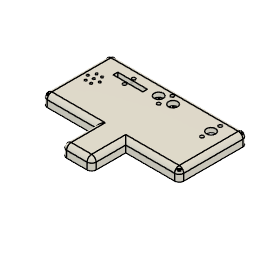
ControllerTopHalf (Autodesk Fusion 360 design; units mm, degrees)
part number: 2026-04-19-10-42-28-781
Autodesk Fusion 360 part; units mm, degrees
sketch "Sketch1" plane through (0, 0, 0) normal (0, 1, 0) x (1, 0, 0)
  line L0 (0, 0) -> (300, 0)
  line L1 (300, 0) -> (300, -150)
  line L2 (300, -150) -> (0, -150)
  line L3 (0, -150) -> (0, 0)
  line L4 (150, -150) -> (117.5, -150)
  line L5 (150, -150) -> (182.5, -150)
  line L6 (117.5, -150) -> (117.5, -225)
  line L7 (182.5, -150) -> (182.5, -225)
  line L8 (117.5, -225) -> (182.5, -225)
  dimension "d1" = 300
  dimension "d2" = 150
  dimension "d3" = 32.5
  dimension "d4" = 32.5
  dimension "d5" = 75
  dimension "d6" = 75
  constraint horizontal L0
  constraint vertical L1
  constraint horizontal L2
  constraint vertical L3
  constraint coincident L0.start L3.end
  constraint midpoint L2 L4.start
  constraint parallel L2 L4
  constraint parallel L2 L5
  constraint perpendicular L2 L6
  constraint perpendicular L2 L7
  measures "d1" distance of L0.start L0.end
  measures "d2" distance of L0.start L2.end
  measures "d3" distance of L4.start L4.end
  measures "d4" distance of L4.start L5.end
  measures "d5" distance of L4.end L6.end
  measures "d6" distance of L5.end L7.end
extrude "Extrude1" add sketch "Sketch1" along normal blind 25
fillet "Fillet1" radius 10 6 edges at (0, 12.5, 0) (0, 12.5, 150) (117.5, 12.5, 225) (182.5, 12.5, 225) (300, 12.5, 150) (300, 12.5, 0) 1 faces at (139.1667, 25, 50)
shell "Shell1" thickness 10 removed faces 1 at (139.1667, 0, 50)
sketch "Sketch2" plane through (0, 25, 0) normal (0, 1, 0) x (-1, 0, 0)
  line L0 (-127.5, 215) -> (-172.5, 215)
  line L1 (-172.5, 215) -> (-172.5, 140)
  line L2 (-172.5, 140) -> (-290, 140)
  line L3 (-290, 140) -> (-290, 10)
  line L4 (-290, 10) -> (-10, 10)
  line L5 (-10, 10) -> (-10, 140)
  line L6 (-10, 140) -> (-127.5, 140)
  line L7 (-127.5, 140) -> (-127.5, 215)
  circle A0 centre (-24.9278, 56.5112) radius 5
  circle A1 centre (-36.9278, 56.5112) radius 5
  circle A2 centre (-17.9278, 68.5112) radius 5
  circle A3 centre (-30.9278, 68.5112) radius 5
  circle A4 centre (-43.9278, 68.5112) radius 5
  circle A5 centre (-24.9278, 80.5112) radius 5
  circle A6 centre (-36.9278, 80.5112) radius 5
  dimension "d12" = 10
  dimension "d13" = 12
  dimension "d14" = 10
  dimension "d17" = 10
  dimension "d19" = 10
  dimension "d22" = 10
  dimension "d25" = 10
  dimension "d26" = 10
  measures "d12" diameter of A0
  measures "d13" distance of A0.centre A1.centre
  measures "d14" diameter of A1
  measures "d17" diameter of A2
  measures "d19" diameter of A3
  measures "d22" diameter of A4
  measures "d25" diameter of A5
  measures "d26" diameter of A6
hole "Hole1" at (17.9278, 25, 68.5112) at (24.9278, 25, 56.5112) at (30.9278, 25, 68.5112) at (36.9278, 25, 56.5112) at (43.9278, 25, 68.5112) at (36.9278, 25, 80.5112) at (24.9278, 25, 80.5112) direction (0, -1, 0) diameter 5 depth 16 tip angle 180
sketch "Sketch3" plane through (0, 25, 0) normal (0, 1, 0) x (-1, 0, 0)
  circle A0 centre (-36.9278, 80.5112) radius 2.5
  circle A1 centre (-36.9278, 56.5112) radius 2.5
  circle A2 centre (-24.9278, 56.5112) radius 2.5
  circle A3 centre (-17.9278, 68.5112) radius 2.5
  circle A4 centre (-30.9278, 68.5112) radius 2.5
  circle A5 centre (-43.9278, 68.5112) radius 2.5
  circle A6 centre (-24.9278, 80.5112) radius 2.5
  line L0 (-127.5, 215) -> (-172.5, 215)
  line L1 (-172.5, 215) -> (-172.5, 140)
  line L2 (-172.5, 140) -> (-290, 140)
  line L3 (-290, 140) -> (-290, 10)
  line L4 (-290, 10) -> (-10, 10)
  line L5 (-10, 10) -> (-10, 140)
  line L6 (-10, 140) -> (-127.5, 140)
  line L7 (-127.5, 140) -> (-127.5, 215)
  circle A7 centre (-260, 40) radius 10
  line L8 (-45, 30) -> (-110, 30)
  line L9 (-110, 30) -> (-110, 40)
  line L10 (-110, 40) -> (-45, 40)
  line L11 (-45, 40) -> (-45, 30)
  dimension "d30" = 20
  constraint horizontal L8
  constraint vertical L9
  constraint horizontal L10
  constraint vertical L11
  measures "d30" diameter of A7
extrude "Extrude2" cut sketch "Sketch3" against normal blind 50 contours A7 | L8 L9 L10 L11
sketch "Sketch4" plane through (0, 25, 0) normal (0, 1, 0) x (-1, 0, 0)
  line L0 (-110, 30) -> (-110, 40)
  line L1 (-110, 40) -> (-45, 40)
  line L2 (-45, 40) -> (-45, 30)
  line L3 (-45, 30) -> (-110, 30)
  circle A0 centre (-260, 40) radius 10
  circle A1 centre (-36.9278, 80.5112) radius 2.5
  circle A2 centre (-36.9278, 56.5112) radius 2.5
  circle A3 centre (-24.9278, 56.5112) radius 2.5
  circle A4 centre (-17.9278, 68.5112) radius 2.5
  circle A5 centre (-30.9278, 68.5112) radius 2.5
  circle A6 centre (-43.9278, 68.5112) radius 2.5
  circle A7 centre (-24.9278, 80.5112) radius 2.5
  line L4 (-127.5, 215) -> (-172.5, 215)
  line L5 (-172.5, 215) -> (-172.5, 140)
  line L6 (-172.5, 140) -> (-290, 140)
  line L7 (-290, 140) -> (-290, 10)
  line L8 (-290, 10) -> (-10, 10)
  line L9 (-10, 10) -> (-10, 140)
  line L10 (-10, 140) -> (-127.5, 140)
  line L11 (-127.5, 140) -> (-127.5, 215)
  circle A8 centre (-135, 30) radius 10
  line L12 (-172.5, 140) -> (-62.5, 140) construction
  circle A9 centre (-166.743, 30.1508) radius 10
  dimension "d33" = 20
  dimension "d36" = 20
  constraint horizontal L12
  constraint coincident L5.end L6.start
  measures "d33" diameter of A8
  measures "d36" diameter of A9
extrude "Extrude3" cut sketch "Sketch4" against normal blind 65 contours A8 | A9
sketch "Sketch5" plane through (0, 25, 0) normal (0, 1, 0) x (-1, 0, 0)
  circle A0 centre (-135, 30) radius 10
  circle A1 centre (-166.743, 30.1508) radius 10
  line L0 (-110, 30) -> (-110, 40)
  line L1 (-110, 40) -> (-45, 40)
  line L2 (-45, 40) -> (-45, 30)
  line L3 (-45, 30) -> (-110, 30)
  circle A2 centre (-260, 40) radius 10
  circle A3 centre (-36.9278, 80.5112) radius 2.5
  circle A4 centre (-36.9278, 56.5112) radius 2.5
  circle A5 centre (-24.9278, 56.5112) radius 2.5
  circle A6 centre (-17.9278, 68.5112) radius 2.5
  circle A7 centre (-30.9278, 68.5112) radius 2.5
  circle A8 centre (-43.9278, 68.5112) radius 2.5
  circle A9 centre (-24.9278, 80.5112) radius 2.5
  line L4 (-127.5, 215) -> (-172.5, 215)
  line L5 (-172.5, 215) -> (-172.5, 140)
  line L6 (-172.5, 140) -> (-290, 140)
  line L7 (-290, 140) -> (-290, 10)
  line L8 (-290, 10) -> (-10, 10)
  line L9 (-10, 10) -> (-10, 140)
  line L10 (-10, 140) -> (-127.5, 140)
  line L11 (-127.5, 140) -> (-127.5, 215)
  circle A10 centre (-75, 45) radius 2
  circle A11 centre (-75, 25) radius 2
  circle A12 centre (-150, 15) radius 2
  circle A13 centre (-150, 45) radius 2
  circle A14 centre (-260, 20) radius 2
  circle A15 centre (-260, 60) radius 2
  dimension "d39" = 4
  dimension "d40" = 4
  dimension "d41" = 4
  dimension "d42" = 4
  dimension "d43" = 4
  dimension "d44" = 4
  measures "d39" diameter of A10
  measures "d40" diameter of A11
  measures "d41" diameter of A12
  measures "d42" diameter of A13
  measures "d43" diameter of A14
  measures "d44" diameter of A15
hole "Hole2" at (150, 25, 45) at (75, 25, 45) at (75, 25, 25) at (150, 25, 15) at (260, 25, 60) at (260, 25, 20) direction (0, -1, 0) diameter 4.234 depth 16 tip angle 180 counterbore diameter 7.5 counterbore depth 5
thread "Thread1" "ISO Metric profile 5.0 M5x0.8 M5x0.8 6H" thread offset 0 thread depth 7.4
sketch "Sketch6" plane through (0, 0, 0) normal (0, -1, 0) x (1, 0, 0)
  line L0 (127.5, 140) -> (127.5, 215)
  line L1 (127.5, 215) -> (172.5, 215)
  line L2 (172.5, 215) -> (172.5, 140)
  line L3 (172.5, 140) -> (290, 140)
  line L4 (290, 140) -> (290, 10)
  line L5 (290, 10) -> (10, 10)
  line L6 (10, 10) -> (10, 140)
  line L7 (10, 140) -> (127.5, 140)
  arc A0 (182.5, 215) -> (172.5, 225) centre (172.5, 215) ccw
  line L8 (172.5, 225) -> (127.5, 225)
  arc A1 (127.5, 225) -> (117.5, 215) centre (127.5, 215) ccw
  line L9 (117.5, 215) -> (117.5, 150)
  line L10 (117.5, 150) -> (10, 150)
  arc A2 (10, 150) -> (0, 140) centre (10, 140) ccw
  line L11 (0, 140) -> (0, 10)
  arc A3 (0, 10) -> (10, 0) centre (10, 10) ccw
  line L12 (10, 0) -> (290, 0)
  arc A4 (290, 0) -> (300, 10) centre (290, 10) ccw
  line L13 (300, 10) -> (300, 140)
  arc A5 (300, 140) -> (290, 150) centre (290, 140) ccw
  line L14 (290, 150) -> (182.5, 150)
  line L15 (182.5, 150) -> (182.5, 215)
sketch "Sketch7" plane through (0, 25, 0) normal (0, 1, 0) x (-1, 0, 0)
  circle A0 centre (-260, 60) radius 3.75
  circle A1 centre (-75, 25) radius 3.75
  circle A2 centre (-150, 45) radius 3.75
  circle A3 centre (-75, 45) radius 3.75
  circle A4 centre (-150, 15) radius 3.75
  circle A5 centre (-260, 20) radius 3.75
  circle A6 centre (-135, 30) radius 10
  circle A7 centre (-166.743, 30.1508) radius 10
  line L0 (-110, 30) -> (-110, 40)
  line L1 (-110, 40) -> (-45, 40)
  line L2 (-45, 40) -> (-45, 30)
  line L3 (-45, 30) -> (-110, 30)
  circle A8 centre (-260, 40) radius 10
  circle A9 centre (-36.9278, 80.5112) radius 2.5
  circle A10 centre (-36.9278, 56.5112) radius 2.5
  circle A11 centre (-24.9278, 56.5112) radius 2.5
  circle A12 centre (-17.9278, 68.5112) radius 2.5
  circle A13 centre (-30.9278, 68.5112) radius 2.5
  circle A14 centre (-43.9278, 68.5112) radius 2.5
  circle A15 centre (-24.9278, 80.5112) radius 2.5
  line L4 (-127.5, 215) -> (-172.5, 215)
  line L5 (-172.5, 215) -> (-172.5, 140)
  line L6 (-172.5, 140) -> (-290, 140)
  line L7 (-290, 140) -> (-290, 10)
  line L8 (-290, 10) -> (-10, 10)
  line L9 (-10, 10) -> (-10, 140)
  line L10 (-10, 140) -> (-127.5, 140)
  line L11 (-127.5, 140) -> (-127.5, 215)
  line L12 (-10, 140) -> (-2.9289, 147.0711)
  line L13 (-10, 10) -> (-2.9289, 2.9289)
  line L14 (-10, 10) -> (0, 10) construction
  line L15 (-290, 10) -> (-297.0711, 2.9289)
  line L16 (-290, 10) -> (-280, 10) construction
  line L17 (-290, 140) -> (-297.0711, 147.0711)
  line L18 (-290, 140) -> (-280, 140) construction
  circle A16 centre (-293.5355, 143.5355) radius 2.116
  circle A17 centre (-293.5355, 6.4645) radius 2.1161
  circle A18 centre (-6.4645, 6.4645) radius 2.116
  circle A19 centre (-6.4645, 143.5355) radius 2.116
  dimension "d52" = 10
  dimension "d53" = 45
  dimension "d54" = 10
  dimension "d55" = 135
  dimension "d56" = 10
  dimension "d57" = 135
  dimension "d58" = 10
  dimension "d59" = 4.232
  dimension "d60" = 4.2322
  dimension "d61" = 4.232
  dimension "d62" = 4.232
  constraint coincident L9.end L10.start
  constraint horizontal L14
  constraint coincident L8.end L9.start
  constraint horizontal L16
  constraint coincident L7.end L8.start
  constraint horizontal L18
  constraint coincident L6.end L7.start
  constraint midpoint L17 A16.centre
  constraint midpoint L15 A17.centre
  constraint midpoint L13 A18.centre
  constraint midpoint L12 A19.centre
  measures "d52" distance of L9.end L12.end
  measures "d53" angle of L13 L14
  measures "d54" distance of L8.end L13.end
  measures "d55" angle of L15 L16
  measures "d56" distance of L7.end L15.end
  measures "d57" angle of L17 L18
  measures "d58" distance of L6.end L17.end
  measures "d59" diameter of A16
  measures "d60" diameter of A17
  measures "d61" diameter of A18
  measures "d62" diameter of A19
hole "Hole3" at (293.5355, 25, 6.4645) at (293.5355, 25, 143.5355) at (6.4645, 25, 143.5355) at (6.4645, 25, 6.4645) direction (0, -1, 0) diameter 4.234 depth 30 tip angle 180 counterbore diameter 7.5 counterbore depth 5
thread "Thread2" "ISO Metric profile 5.0 M5x0.8 M5x0.8 6H" thread offset 0 thread depth 7.4
sketch "Sketch8" plane through (0, 0, 0) normal (0, 0, -1) x (-1, 0, 0)
  line L0 (-290, 15) -> (-290, 0)
  line L1 (-290, 0) -> (-10, 0)
  line L2 (-10, 0) -> (-10, 15)
  line L3 (-10, 15) -> (-290, 15)
  line L4 (-10, 15) -> (-75, 15)
  line L5 (-75, 15) -> (-75, 3)
  line L6 (-75, 3) -> (-75, 0)
  circle A0 centre (-75, 0) radius 5
  dimension "d70" = 12
  dimension "d71" = 10
  constraint coincident L2.end L3.start
  constraint coincident L3 L4.end
  constraint perpendicular L4 L5
  constraint coincident L1 L6.end
  constraint perpendicular L1 L6
  constraint coincident L6.end A0.centre
  measures "d70" distance of L4.end L5.end
  measures "d71" diameter of A0
extrude "Extrude4" cut sketch "Sketch8" against normal blind 26 contours L1 L5 L6 A0 | L1 L5 L6 A0
sketch "Sketch9" plane through (0, 0, 0) normal (0, 0, -1) x (-1, 0, 0)
  arc A0 (-70, 0) -> (-80, 0) centre (-75, 0) ccw
  line L0 (-70, 0) -> (-10, 0)
  line L1 (-10, 0) -> (-10, 15)
  line L2 (-10, 15) -> (-290, 15)
  line L3 (-290, 15) -> (-290, 0)
  line L4 (-290, 0) -> (-230, 0)
  circle A1 centre (-230, 0) radius 5
  line L5 (-225, 0) -> (-218, 0)
  circle A2 centre (-218, 0) radius 5
  line L6 (-213, 0.0203) -> (-206, 0.0203)
  circle A3 centre (-206, 0.0203) radius 5
  dimension "d79" = 60
  dimension "d80" = 10
  dimension "d81" = 7
  dimension "d82" = 10
  dimension "d83" = 7
  dimension "d84" = 10
  constraint coincident L3.end L4.start
  constraint perpendicular L3 L4
  constraint coincident L4.end A1.centre
  constraint coincident A1 L5.start
  constraint horizontal L5
  constraint coincident L5.end A2.centre
  constraint coincident A2 L6.start
  constraint horizontal L6
  constraint coincident L6.end A3.centre
  measures "d79" distance of L3.end L4.end
  measures "d80" diameter of A1
  measures "d81" distance of L5.start L5.end
  measures "d82" diameter of A2
  measures "d83" distance of L6.start L6.end
  measures "d84" diameter of A3
sketch "Sketch10" plane through (0, 0, 0) normal (0, 0, -1) x (-1, 0, 0)
  arc A0 (-70, 0) -> (-80, 0) centre (-75, 0) ccw
  line L0 (-70, 0) -> (-10, 0)
  line L1 (-10, 0) -> (-10, 15)
  line L2 (-10, 15) -> (-290, 15)
  line L3 (-290, 15) -> (-290, 0)
  line L4 (-290, 0) -> (-80, 0)
  line L5 (-290, 0) -> (-230, 0)
  line L6 (-230, 0) -> (-225, 0)
  circle A1 centre (-225, 0) radius 5
  line L7 (-220, 0) -> (-213, 0)
  circle A2 centre (-213, 0) radius 5
  line L8 (-208, 0) -> (-201, 0)
  circle A3 centre (-201, 0) radius 5
  dimension "d85" = 60
  dimension "d86" = 5
  dimension "d87" = 10
  dimension "d88" = 7
  dimension "d89" = 10
  dimension "d90" = 7
  dimension "d91" = 10
  constraint coincident L3.end L4.start
  constraint perpendicular L3 L5
  constraint parallel L4 L6
  constraint coincident L6.end A1.centre
  constraint coincident A1 L7.start
  constraint coincident L4 L7.start
  constraint parallel L4 L7
  constraint coincident L7.end A2.centre
  constraint coincident L4 L8.start
  constraint coincident A2 L8.start
  constraint parallel L4 L8
  constraint coincident L8.end A3.centre
  measures "d85" distance of L3.end L5.end
  measures "d86" distance of L5.end L6.end
  measures "d87" diameter of A1
  measures "d88" distance of L7.start L7.end
  measures "d89" diameter of A2
  measures "d90" distance of L8.start L8.end
  measures "d91" diameter of A3
extrude "Extrude5" cut sketch "Sketch10" against normal blind 30 contours L4 L8 A3 | L4 L7 A2 | L4 L6 A1 picked at (-204.3147, 0.2484) picked at (-216.3147, 0.2484) picked at (-223.5578, 2.9948)
